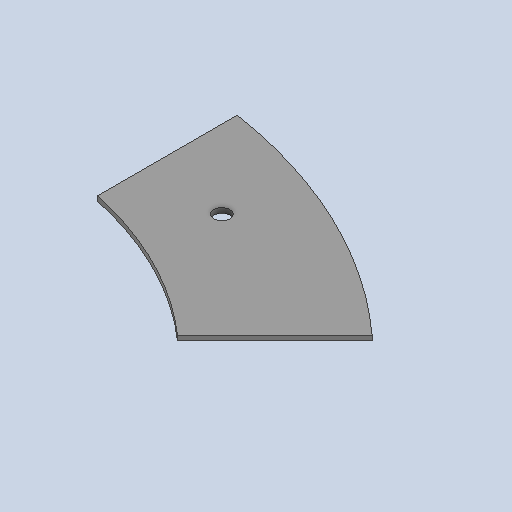
# Autodesk Inventor part: Battery Module Third Iteration
Saved by Autodesk Inventor 2023 (Build 270158000, 158)
## iProperties
Created: 2023-03-05
Part Number: Battery Module Third Iteration
Material: PLA Plastic
Document SubType Name: Modeling
Designer: mihal
Density: 1.25002 g/cm^3
Appearance: Generic
Mass: 46.201 g
Surface Area: 261.24 cm^2
Volume: 36.9601 cm^3
Author: mihal
Autodesk Inventor part; units mm, degrees
ref_plane "YZ Plane" through (0, 0, 0) normal (1, 0, 0) x (0, 1, 0)
ref_plane "XZ Plane" through (0, 0, 0) normal (0, 1, 0) x (-1, 0, 0)
ref_plane "XY Plane" through (0, 0, 0) normal (0, 0, 1) x (1, 0, 0)
sketch "Sketch1" plane through (0, 0, 0) normal (0, 1, 0) x (-1, 0, 0)
  circle A0 centre (0, 0) radius 215
  circle A1 centre (0, 0) radius 315
  line L0 (0, 0) -> (0, -315)
  line L1 (0, 0) -> (-222.7386, -222.7386)
  line L2 (-141.0509, -162.2641) -> (-211.8794, -233.0926)
  line L3 (-15, -214.4761) -> (-15, -314.6427)
  circle A2 centre (0, 0) radius 222.5
  circle A3 centre (0, 0) radius 307.5
  line L4 (-47, -311.4739) -> (-47, -209.7999)
  point P0 (-152.028, -152.028)
  point P1 (0, -215)
  point P2 (0, -312.5)
  point P3 (0, -217.5)
  point P4 (-153.7957, -153.7957)
  point P5 (-220.9709, -220.9709)
  point P6 (-210.1096, -231.3228)
  point P7 (-15, -312.1398)
  point P8 (-15, -216.9821)
  point P9 (-142.8229, -164.0361)
  point P10 (-206.5699, -227.7831)
  point P11 (-15, -307.1339)
  point P12 (-15, -221.9938)
  point P13 (-146.3667, -167.5799)
  point P14 (-47, -303.8869)
  point P15 (-47, -217.4793)
  dimension "d2" = 430
  dimension "d3" = 630
  dimension "d4" = 45
  dimension "d5" = 15
  dimension "d6" = 15
  dimension "d11" = 7.5
  dimension "d12" = 7.5
  dimension "d16" = 32
  constraints: 10 end point, 8 point on circle, 4 centre point, 4 coincident, 3 parallel, 2 vertical
  measures "d2" diameter of A0
  measures "d3" diameter of A1
  measures "d4" angle of L1 L0
  measures "d5" distance between parallel lines of L2 L1
  measures "d6" distance between parallel lines of L3 L0
  measures "d11" radial gap between concentric circles of A0 A2
  measures "d12" radial gap between concentric circles of A3 A1
  measures "d16" distance between parallel lines of L4 L3
extrude "Extrusion1" add sketch "Sketch1" along normal blind 3 contours A2 L4 A3 L2 | A2 L3 A3 L4
sketch "Sketch4" plane through (0, 0, 0) normal (0, 0, 1) x (1, 0, 0)
  line L0 (15, 0) -> (146.3667, 0) projected
  line L1 (146.3667, 0) -> (146.3667, 3) projected
  line L2 (15, 3) -> (146.3667, 3) projected
  line L3 (15, 0) -> (15, 3) projected
  line L4 (15, 0) -> (47, 0)
  line L5 (47, 0) -> (47, 3)
  line L6 (47, 3) -> (15, 3)
  line L7 (15, 3) -> (15, 0)
  point P0 (0, 0)
  dimension "d17" = 32
  constraints: 8 end point, 2 parallel, 1 horizontal, 1 perpendicular, 1 point on line
  measures "d17" distance of L6.end L5.end
extrude "Extrusion3" cut sketch "Sketch4" against normal up to surface contours L3 L2 L5 L0
sketch "Sketch5" plane through (0, 3, 0) normal (0, 1, 0) x (1, 0, 0)
  line L0 (47, 303.8869) -> (47, 217.4793) projected
  arc A0 (146.3667, 167.5799) -> (47, 217.4793) centre (0, 0) ccw projected
  line L1 (146.3667, 167.5799) -> (206.5699, 227.7831) projected
  arc A1 (206.5699, 227.7831) -> (47, 303.8869) centre (0, 0) ccw projected
  line L2 (146.3667, 167.5799) -> (206.5699, 227.7831) projected
  line L3 (47, 217.4793) -> (47, 303.8869) projected
  circle A2 centre (50, 219.8092) radius 1.75
  circle A3 centre (143.9011, 173.5996) radius 1.75
  circle A4 centre (199.96, 229.6585) radius 1.75
  circle A5 centre (50, 300.4077) radius 1.75
  arc A6 (146.3667, 167.5799) -> (47, 217.4793) centre (0, 0) ccw projected
  line L4 (99.8507, 198.8368) -> (132.3721, 277.5498) construction
  arc A7 (206.5699, 227.7831) -> (47, 303.8869) centre (0, 0) ccw projected
  line L5 (116.1114, 238.1933) -> (47, 266.7477) construction
  line L6 (116.1114, 238.1933) -> (187.4893, 208.7025) construction
  line L7 (50, 300.4077) -> (50, 298.6577) construction
  line L8 (50, 300.4077) -> (47, 300.4077) construction
  line L9 (143.9011, 173.5996) -> (148.1437, 169.3569) construction
  line L10 (50, 219.8092) -> (47, 219.8092) construction
  line L11 (199.96, 229.6585) -> (204.2027, 225.4159) construction
  line L12 (50, 216.8092) -> (50, 303.4077) construction
  line L13 (141.7806, 171.4774) -> (202.1185, 231.742) construction
  dimension "d36" = 3.5
  dimension "d37" = 3
  dimension "d40" = 3.5
  dimension "d45" = 6
  dimension "d47" = 3.5
  dimension "d48" = 3.5
  dimension "d49" = 6
  dimension "d51" = 3
  dimension "d53" = 3
  dimension "d54" = 3
  dimension "d55" = 3
  dimension "d56" = 3
  constraints: 20 end point, 8 point on circle, 6 perpendicular, 6 point on line, 3 centre point, 3 vertical, 1 midpoint, 1 vertical alignment, 3 other
  measures "d37" distance of L7.start L8.end
  measures "d40" diameter of A2
  measures "d45" distance of L9.start L9.end
  measures "d47" diameter of A4
  measures "d48" diameter of A3
  measures "d49" distance of L11.start L11.end
  measures "d51" distance of L10.start L10.end
  measures "d53" distance of L12.end L7.start
  measures "d54" distance of L12.start L10.start
  measures "d55" distance of L13.start L9.start
  measures "d56" distance of L13.end L11.start
extrude "Extrusion4" [suppressed]
sketch "Sketch6" plane through (0, 3, 0) normal (0, 1, 0) x (1, 0, 0)
  line L0 (47, 303.8869) -> (47, 217.4793) projected
  arc A0 (146.3667, 167.5799) -> (47, 217.4793) centre (0, 0) ccw projected
  line L1 (146.3667, 167.5799) -> (206.5699, 227.7831) projected
  arc A1 (206.5699, 227.7831) -> (47, 303.8869) centre (0, 0) ccw projected
  line L2 (0, 0) -> (132.3721, 277.5498)
  arc A2 (206.5699, 227.7831) -> (47, 303.8869) centre (0, 0) ccw projected
  arc A3 (146.3667, 167.5799) -> (47, 217.4793) centre (0, 0) ccw projected
  line L3 (95.7814, 200.8287) -> (132.3721, 277.5498)
  line L4 (114.0768, 239.1892) -> (95.7814, 200.8287)
  line L5 (146.3667, 167.5799) -> (206.5699, 227.7831) projected
  line L6 (176.4683, 197.6815) -> (47, 260.6831)
  line L7 (47, 217.4793) -> (47, 303.8869) projected
  circle A4 centre (95.3, 246.0764) radius 5
  point P0 (104.9291, 220.009)
  dimension "d61" = 10
  dimension "d62" = 20
  dimension "d63" = 8
  constraints: 8 end point, 4 midpoint, 3 point on circle, 1 centre point, 1 coincident, 1 collinear, 1 point on line
  measures "d61" diameter of A4
  measures "d62" distance of point (114.077, 239.189) A4.centre
  measures "d63" distance from line of L6 A4.centre
extrude "Extrusion5" cut sketch "Sketch6" against normal blind 10 contours A4
body "Solid1"
